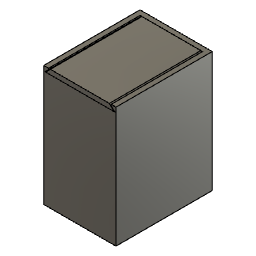
box sliding top v2 (Autodesk Fusion 360 design; units mm, degrees)
Autodesk Fusion 360 part; units mm, degrees
note: some values were not read from the file. Set by a fixed rule: which face or edge a step refers to.
sketch "Sketch1" plane through (0, 0, 0) normal (0, 1, 0) x (1, 0, 0)
  line L0 (38.1, -50.8) -> (-38.1, -50.8)
  line L1 (-38.1, -50.8) -> (-38.1, 50.8)
  line L2 (-38.1, 50.8) -> (38.1, 50.8)
  line L3 (38.1, 50.8) -> (38.1, -50.8)
  line L4 (38.1, -50.8) -> (-38.1, 50.8) construction
  line L5 (-38.1, -50.8) -> (38.1, 50.8) construction
  dimension "d1" = 76.2
  dimension "d2" = 101.6
  constraint horizontal L0
  constraint perpendicular L0 L1
  constraint parallel L0 L2
  constraint parallel L1 L3
  constraint coincident L4 origin
  constraint coincident L5 origin
  measures "d1" distance of L1.end L2.end
  measures "d2" distance of L0.end L1.end
extrude "Extrude1" add sketch "Sketch1" along normal blind 127 makes body 1
shell "Shell1" thickness 5.08 removed faces 1 at (12.7, 127, 16.9333) on bodies 1
sketch "Sketch2" plane through (0, 0, 50.8) normal (0, 0, 1) x (1, 0, 0)
  line L0 (-38.1, 0) -> (38.1, 0)
  line L1 (38.1, 0) -> (38.1, 127)
  line L2 (38.1, 127) -> (-38.1, 127)
  line L3 (-38.1, 127) -> (-38.1, 0)
  line L4 (-33.02, 5.08) -> (-33.02, 127)
  line L5 (-33.02, 127) -> (-33.02, 5.08)
  line L6 (33.02, 5.08) -> (33.02, 127)
  line L7 (33.02, 127) -> (33.02, 5.08)
  line L8 (-38.1, 121.92) -> (38.1, 121.92)
  line L9 (-36.83, 121.92) -> (-33.02, 125.73)
  line L10 (0, 2.5) -> (0, 20)
  line L11 (36.83, 121.92) -> (33.02, 125.73)
  dimension "d6" = 5.08
  dimension "d7" = 1.27
  constraint coincident L3 L8.start
  constraint coincident L1 L8.end
  constraint perpendicular L1 L8
  constraint coincident L8 L9.start
  constraint coincident L4 L9.end
  constraint symmetric L9.start L10 L11.start
  constraint symmetric L9.end L10 L11.end
  measures "d6" distance of L2 L8
  measures "d7" distance of L4.end L9.end
extrude "Extrude2" cut sketch "Sketch2" against normal up to surface (96.52 mm away) contours L4 L5 L8 L9 | L6 L7 L8 L11 | L2 L4 L5 L6 L7 L8 bodies 1
sketch "Sketch1 (2)" plane through (0, 0, 50.8) normal (0, 0, 1) x (1, 0, 0) in component "Component"
  line L0 (-33.02, 125.73) -> (-33.02, 127)
  line L1 (-33.02, 127) -> (-38.1, 127)
  line L2 (-38.1, 127) -> (-38.1, 0)
  line L3 (-38.1, 0) -> (38.1, 0)
  line L4 (38.1, 0) -> (38.1, 127)
  line L5 (38.1, 127) -> (33.02, 127)
  line L6 (33.02, 127) -> (33.02, 125.73)
  line L7 (33.02, 125.73) -> (36.83, 121.92)
  line L8 (36.83, 121.92) -> (-36.83, 121.92)
  line L9 (-36.83, 121.92) -> (-33.02, 125.73)
  line L10 (-33.02, 125.73) -> (-31.82, 126.93)
  line L11 (33.02, 125.73) -> (31.82, 126.93)
  line L12 (31.82, 126.93) -> (-31.82, 126.93)
  constraint coincident L0.start L9.end
  constraint coincident L6.end L7.start
  constraint parallel L9 L10
  constraint parallel L7 L11
  constraint horizontal L12
extrude "Extrude1'" add sketch "Sketch1 (2)" against normal up to surface (96.52 mm away) separate body contours L7 L8 L9 L10 L11 L12 makes body 2 in component "Component"
move_face "OffsetFaces1" offset -0.508 4 faces at (-32.62, 126.13, -13.5467) (-35.56, 123.19, 18.6267) (32.62, 126.13, 18.6267) (34.29, 124.46, 18.6267) on bodies 2 in component "Component"
fillet "Fillet1" radius 0.254 2 edges at (-36.1116, 121.92, 2.54) (36.1116, 121.92, 2.54) on bodies 2 in component "Component"
component "Component" placed x (1, 0, 0) y (0, 1, 0) z (0, 0, 1) at (0, 0, 0)
